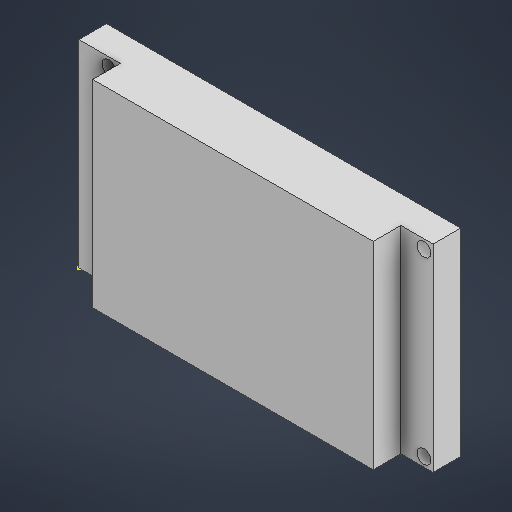
# Autodesk Inventor part: Pantalla
Saved by Autodesk Inventor 2026 (Build 300175000, 175)
## iProperties
Created: 2026-04-21
Part Number: Pantalla
Material: Generic
Document SubType Name: Modeling
Designer: juana
Density: 1 g/cm^3
Appearance: Default
Author: juana
Autodesk Inventor part; units mm, degrees
ref_plane "YZ Plane" through (0, 0, 0) normal (1, 0, 0) x (0, 1, 0)
ref_plane "XZ Plane" through (0, 0, 0) normal (0, 1, 0) x (-1, 0, 0)
ref_plane "XY Plane" through (0, 0, 0) normal (0, 0, 1) x (1, 0, 0)
sketch "Sketch1" plane through (0, 0, 0) normal (0, 0, 1) x (1, 0, 0)
  line L0 (0, 43) -> (77, 43)
  line L1 (77, 43) -> (77, 0)
  line L2 (77, 0) -> (0, 0)
  line L3 (0, 0) -> (0, 43)
  point P0 (74.8142, 2.33)
  point P1 (74.8142, 51.9717)
  dimension "d0" = 77
  dimension "d1" = 43
  constraints: 8 end point, 2 parallel, 2 vertical alignment, 1 horizontal, 1 horizontal alignment, 1 perpendicular
  measures "d0" distance of L1.end L2.end
  measures "d1" distance of L2.end L0.start
extrude "Extrusion1" add sketch "Sketch1" along normal blind 6
sketch "Sketch2" plane through (0, 0, 6) normal (0, 0, 1) x (1, 0, 0)
  point P0 (0, 0)
sketch "Sketch3" plane through (0, 0, 6) normal (0, 0, 1) x (1, 0, 0)
  line L0 (9, 43) -> (70, 43)
  line L1 (70, 43) -> (70, 0)
  line L2 (70, 0) -> (9, 0)
  line L3 (9, 0) -> (9, 43)
  line L4 (77, 0) -> (77, 43) projected
  line L5 (0, 0) -> (77, 0) projected
  line L6 (77, 43) -> (0, 43) projected
  point P0 (75, 41)
  point P1 (75, 2)
  dimension "d4" = 61
  dimension "d5" = 7
  dimension "d6" = 2
  dimension "d7" = 2
  dimension "d8" = 2
  constraints: 8 end point, 2 horizontal alignment, 2 parallel, 1 horizontal, 1 perpendicular, 1 vertical alignment
  measures "d4" distance of L0.start L0.end
  measures "d5" distance between parallel lines of L4 L1
  measures "d6" distance from line of L4 point (75, 2)
  measures "d7" distance from line of L5 point (75, 2)
  measures "d8" distance from line of L6 point (75, 41)
extrude "Extrusion2" add sketch "Sketch3" along normal blind 6 contours L0 L1 L2 L3
sketch "Sketch4" plane through (0, 0, 6) normal (0, 0, 1) x (1, 0, 0)
  line L0 (77, 43) -> (70, 43) projected
  line L1 (70, 0) -> (77, 0) projected
  line L2 (77, 0) -> (77, 43) projected
  point P0 (0, 0)
  point P1 (75, 2)
  point P2 (75, 41)
  dimension "d11" = 2
  dimension "d12" = 2
  dimension "d13" = 2
  constraints: 1 vertical alignment
  measures "d11" distance from line of L0 point (75, 41)
  measures "d12" distance from line of point (75, 2) L1
  measures "d13" distance from line of L2 point (75, 2)
hole "Hole1" at (75, 2, 6) at (75, 41, 6) direction (0, 0, -1) diameter 3 end through all
sketch "Sketch5" plane through (0, 0, 6) normal (0, 0, 1) x (1, 0, 0)
  line L0 (9, 43) -> (0, 43) projected
  line L1 (0, 0) -> (9, 0) projected
  line L2 (0, 43) -> (0, 0) projected
  point P0 (6.5, 2)
  point P1 (6.5, 41)
  dimension "d21" = 2
  dimension "d22" = 2
  dimension "d23" = 6.5
  constraints: 1 vertical alignment
  measures "d21" distance from line of L0 point (6.5, 41)
  measures "d22" distance from line of L1 point (6.5, 2)
  measures "d23" distance from line of L2 point (6.5, 41)
hole "Hole2" at (6.5, 41, 6) at (6.5, 2, 6) direction (0, 0, -1) diameter 3 end through all
body "Solid1"
